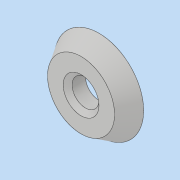
# Autodesk Inventor part: SpurGearThrustDistributer
Saved by Autodesk Inventor 2017 (Build 210142000, 142)
## iProperties
Created: 2016-11-28
Part Number: SpurGearThrustDistributer
Material: Generic
Document SubType Name: Modeling
Designer: techn
Density: 1 g/cm^3
Appearance: Default
Author: techn
Autodesk Inventor part; units mm, degrees
ref_plane "YZ Plane" through (0, 0, 0) normal (1, 0, 0) x (0, 1, 0)
ref_plane "XZ Plane" through (0, 0, 0) normal (0, 1, 0) x (-1, 0, 0)
ref_plane "XY Plane" through (0, 0, 0) normal (0, 0, 1) x (1, 0, 0)
sketch "Sketch2" plane through (0, 0, 0) normal (0, 0, 1) x (1, 0, 0)
  circle A0 centre (0, 0) radius 4.7625
  circle A1 centre (0, 0) radius 15.875
  dimension "d3" = 9.525
  dimension "d4" = 31.75
  constraints: 2 centre point, 2 coincident
  measures "d3" diameter of A0
  measures "d4" diameter of A1
extrude "Extrusion2" add sketch "Sketch2" along normal blind 6.35
sketch "Sketch3" plane through (0, 0, 0) normal (0, 0, -1) x (-1, 0, 0)
  line L0 (0, 0) -> (0, 9.2207)
  circle A0 centre (0, 9.2207) radius 3.81
  circle A1 centre (-7.9854, -4.6104) radius 3.81
  circle A2 centre (7.9854, -4.6104) radius 3.81
  dimension "d7" = 7.62
  dimension "d10" = 360
  constraints: 3 centre point, 2 end point, 1 coincident, 1 vertical, 7 other
  measures "d7" diameter of A0
extrude "Extrusion3" cut sketch "Sketch3" against normal blind 3.175
chamfer "Chamfer1" distance 1.5875 angle 45 1 edges at (-4.7625, 0, 6.35)
chamfer "Chamfer2" distance 3.9688 distance2 6.35 1 edges at (-15.875, 0, 6.35) measured on face at (-15.375, 0, 6.35)
body "Solid2"
